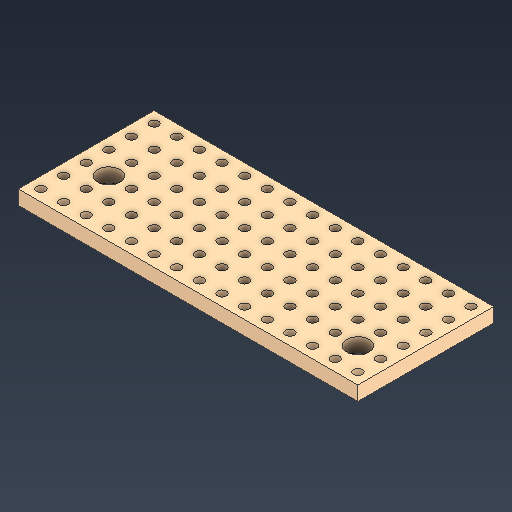
# Autodesk Inventor part: Board
Saved by Autodesk Inventor 2021 (Build 250183000, 183)
## iProperties
Created: 2021-01-22
Part Number: Board
Material: Generic
Document SubType Name: Modeling
Designer: User
Density: 1 g/cm^3
Appearance: Default
Author: User
Autodesk Inventor part; units mm, degrees
ref_plane "YZ Plane" through (0, 0, 0) normal (1, 0, 0) x (0, 1, 0)
ref_plane "XZ Plane" through (0, 0, 0) normal (0, 1, 0) x (-1, 0, 0)
ref_plane "XY Plane" through (0, 0, 0) normal (0, 0, 1) x (1, 0, 0)
sketch "Sketch1" plane through (0, 0, 0) normal (0, 1, 0) x (-1, 0, 0)
  line L0 (19.05, -7.62) -> (-19.05, -7.62)
  line L1 (-19.05, -7.62) -> (-19.05, 7.62)
  line L2 (-19.05, 7.62) -> (19.05, 7.62)
  line L3 (19.05, 7.62) -> (19.05, -7.62)
  line L4 (19.05, -7.62) -> (-19.05, 7.62) construction
  line L5 (-19.05, -7.62) -> (19.05, 7.62) construction
  circle A0 centre (17.78, -6.35) radius 0.5
  circle A1 centre (15.24, -6.35) radius 0.5
  circle A2 centre (12.7, -6.35) radius 0.5
  circle A3 centre (10.16, -6.35) radius 0.5
  circle A4 centre (7.62, -6.35) radius 0.5
  circle A5 centre (5.08, -6.35) radius 0.5
  circle A6 centre (2.54, -6.35) radius 0.5
  circle A7 centre (0, -6.35) radius 0.5
  circle A8 centre (17.78, -3.81) radius 0.5
  circle A9 centre (15.24, -3.81) radius 0.5
  circle A10 centre (12.7, -3.81) radius 0.5
  circle A11 centre (10.16, -3.81) radius 0.5
  circle A12 centre (7.62, -3.81) radius 0.5
  circle A13 centre (5.08, -3.81) radius 0.5
  circle A14 centre (2.54, -3.81) radius 0.5
  circle A15 centre (0, -3.81) radius 0.5
  circle A16 centre (17.78, -1.27) radius 0.5
  circle A17 centre (15.24, -1.27) radius 0.5
  circle A18 centre (12.7, -1.27) radius 0.5
  circle A19 centre (10.16, -1.27) radius 0.5
  circle A20 centre (7.62, -1.27) radius 0.5
  circle A21 centre (5.08, -1.27) radius 0.5
  circle A22 centre (2.54, -1.27) radius 0.5
  circle A23 centre (0, -1.27) radius 0.5
  circle A24 centre (-2.54, -6.35) radius 0.5
  circle A25 centre (-2.54, -3.81) radius 0.5
  circle A26 centre (-2.54, -1.27) radius 0.5
  circle A27 centre (-5.08, -6.35) radius 0.5
  circle A28 centre (-5.08, -3.81) radius 0.5
  circle A29 centre (-5.08, -1.27) radius 0.5
  circle A30 centre (17.78, 1.27) radius 0.5
  circle A31 centre (15.24, 1.27) radius 0.5
  circle A32 centre (12.7, 1.27) radius 0.5
  circle A33 centre (10.16, 1.27) radius 0.5
  circle A34 centre (7.62, 1.27) radius 0.5
  circle A35 centre (5.08, 1.27) radius 0.5
  circle A36 centre (2.54, 1.27) radius 0.5
  circle A37 centre (0, 1.27) radius 0.5
  circle A38 centre (-2.54, 1.27) radius 0.5
  circle A39 centre (-5.08, 1.27) radius 0.5
  circle A40 centre (-7.62, -6.35) radius 0.5
  circle A41 centre (-7.62, -3.81) radius 0.5
  circle A42 centre (-7.62, -1.27) radius 0.5
  circle A43 centre (-7.62, 1.27) radius 0.5
  circle A44 centre (-10.16, -6.35) radius 0.5
  circle A45 centre (-10.16, -3.81) radius 0.5
  circle A46 centre (-10.16, -1.27) radius 0.5
  circle A47 centre (-10.16, 1.27) radius 0.5
  circle A48 centre (-12.7, -6.35) radius 0.5
  circle A49 centre (-12.7, -3.81) radius 0.5
  circle A50 centre (-12.7, -1.27) radius 0.5
  circle A51 centre (-12.7, 1.27) radius 0.5
  circle A52 centre (-15.24, -6.35) radius 0.5
  circle A53 centre (-15.24, -3.81) radius 0.5
  circle A54 centre (-15.24, -1.27) radius 0.5
  circle A55 centre (-15.24, 1.27) radius 0.5
  circle A56 centre (-17.78, -6.35) radius 0.5
  circle A57 centre (-17.78, -3.81) radius 0.5
  circle A58 centre (-17.78, -1.27) radius 0.5
  circle A59 centre (-17.78, 1.27) radius 0.5
  circle A60 centre (17.78, 3.81) radius 0.5
  circle A61 centre (15.24, 3.81) radius 0.5
  circle A62 centre (12.7, 3.81) radius 0.5
  circle A63 centre (10.16, 3.81) radius 0.5
  circle A64 centre (7.62, 3.81) radius 0.5
  circle A65 centre (5.08, 3.81) radius 0.5
  circle A66 centre (2.54, 3.81) radius 0.5
  circle A67 centre (0, 3.81) radius 0.5
  circle A68 centre (-2.54, 3.81) radius 0.5
  circle A69 centre (-5.08, 3.81) radius 0.5
  circle A70 centre (-7.62, 3.81) radius 0.5
  circle A71 centre (-10.16, 3.81) radius 0.5
  circle A72 centre (-12.7, 3.81) radius 0.5
  circle A73 centre (-15.24, 3.81) radius 0.5
  circle A74 centre (-17.78, 3.81) radius 0.5
  circle A75 centre (17.78, 6.35) radius 0.5
  circle A76 centre (15.24, 6.35) radius 0.5
  circle A77 centre (12.7, 6.35) radius 0.5
  circle A78 centre (10.16, 6.35) radius 0.5
  circle A79 centre (7.62, 6.35) radius 0.5
  circle A80 centre (5.08, 6.35) radius 0.5
  circle A81 centre (2.54, 6.35) radius 0.5
  circle A82 centre (0, 6.35) radius 0.5
  circle A83 centre (-2.54, 6.35) radius 0.5
  circle A84 centre (-5.08, 6.35) radius 0.5
  circle A85 centre (-7.62, 6.35) radius 0.5
  circle A86 centre (-10.16, 6.35) radius 0.5
  circle A87 centre (-12.7, 6.35) radius 0.5
  circle A88 centre (-15.24, 6.35) radius 0.5
  circle A89 centre (-17.78, 6.35) radius 0.5
  point P0 (0, 0)
  dimension "d0" = 38.1
  dimension "d1" = 15.24
  dimension "d2" = 1
  dimension "d5" = 2.54
  dimension "d8" = 2.54
  dimension "d11" = 1.27
  dimension "d12" = 1.27
  constraints: 90 centre point, 12 end point, 2 horizontal, 2 midpoint, 2 parallel, 1 perpendicular, 1 vertical, 178 other
  measures "d0" distance of L1.end L2.end
  measures "d1" distance of L0.end L1.end
  measures "d2" diameter of A0
  measures "d5" distance of A0.centre A1.centre
  measures "d8" distance of A0.centre A8.centre
  measures "d11" distance from line of L0 A0.centre
  measures "d12" distance from line of L3 A0.centre
extrude "Extrusion1" add sketch "Sketch1" along normal blind 1.6
sketch "Sketch3" plane through (0, 1.6, 0) normal (0, 1, 0) x (1, 0, 0)
  circle A0 centre (-15.24, -1.27) radius 1.25
  circle A1 centre (15.24, -3.81) radius 1.25
  line L0 (-19.05, 7.62) -> (-19.05, -7.62) projected
  line L1 (19.05, -7.62) -> (19.05, 7.62) projected
  line L2 (19.05, 7.62) -> (-19.05, 7.62) projected
  point P0 (0, 0)
  dimension "d15" = 2.5
  dimension "d16" = 2.5
  dimension "d17" = 3.81
  dimension "d18" = 3.81
  dimension "d19" = 8.89
  dimension "d20" = 11.43
  constraints: 2 centre point
  measures "d15" diameter of A0
  measures "d16" diameter of A1
  measures "d17" distance from line of L0 A0.centre
  measures "d18" distance from line of L1 A1.centre
  measures "d19" distance from line of L2 A0.centre
  measures "d20" distance from line of L2 A1.centre
extrude "Extrusion2" cut sketch "Sketch3" against normal up to surface (1.6 mm away)
equation "\"d0\" = 2.54 * cols"
equation "\"d1\" = 2.54 * rows"
equation "\"d18\" = d17"
equation "\"cols\" = 15"
equation "\"rows\" = 6"
body "Solid1"
